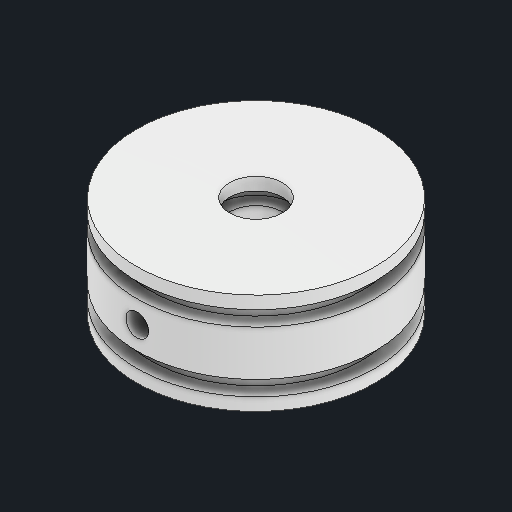
# Autodesk Inventor part: WashPiston_1
Saved by Autodesk Inventor 2024 (Build 280153000, 153)
## iProperties
Created: 2025-02-07
Part Number: WashPiston_1
Material: PVC-Piping
Document SubType Name: Modeling
Designer: Tommy Rohmann
Density: 1.4 g/cm^3
Appearance: Smooth - White
Author: Tommy Rohmann
Autodesk Inventor part; units mm, degrees
ref_plane "YZ Plane" through (0, 0, 0) normal (1, 0, 0) x (0, 1, 0)
ref_plane "XZ Plane" through (0, 0, 0) normal (0, 1, 0) x (-1, 0, 0)
ref_plane "XY Plane" through (0, 0, 0) normal (0, 0, 1) x (1, 0, 0)
sketch "WashPiston" plane through (0, 0, 0) normal (0, 0, 1) x (1, 0, 0)
  line L0 (53.5946, 10.152) -> (53.5946, 15.486)
  line L1 (53.5946, 15.486) -> (47.8796, 15.486)
  line L2 (47.8796, 15.486) -> (47.8796, 21.836)
  line L3 (47.8796, 21.836) -> (53.5946, 21.836)
  line L4 (53.5946, 21.836) -> (53.5946, 40.886)
  line L5 (53.5946, 40.886) -> (47.8796, 40.886)
  line L6 (47.8796, 40.886) -> (47.8796, 47.236)
  line L7 (47.8796, 47.236) -> (53.5946, 47.236)
  line L8 (53.5946, 47.236) -> (53.5946, 52.57)
  line L9 (54.2296, 29.069) -> (54.2296, 79.2986)
  line L10 (3.4296, 2.2226) -> (3.4296, 64.1408)
  line L11 (53.5946, 10.152) -> (3.4296, 10.152)
  line L12 (3.4296, 52.57) -> (53.5946, 52.57)
  line L13 (3.4296, 52.57) -> (3.4296, 10.152)
  line L14 (14.5421, 47.236) -> (19.8761, 47.236)
  line L15 (19.8761, 47.236) -> (19.8761, 41.902)
  line L16 (19.8761, 41.902) -> (14.5421, 41.902)
  line L17 (14.5421, 21.836) -> (3.4296, 21.836)
  line L18 (14.5421, 52.57) -> (14.5421, 47.236)
  line L19 (14.5421, 41.902) -> (14.5421, 21.836)
  point P0 (34.2963, 101.758)
  dimension "d94" = 0.635
  dimension "d95" = 6.35
  dimension "d97" = 6.35
  dimension "d98" = 19.05
  dimension "d99" = 6.35
  dimension "d100" = 5.334
  dimension "d101" = 5.334
  dimension "d103" = 5.334
  dimension "d105" = 101.6
  dimension "d108" = 22.225
  dimension "d141" = 0
  dimension "d142" = 5.334
  dimension "WashPistonHeight" = 42.418
  dimension "d431" = 30.734
  measures "d94" distance between parallel lines of L0 L9
  measures "d95" distance between parallel lines of L7 L5
  measures "d97" distance between parallel lines of L9 L6
  measures "d98" distance of L3.end L4.end
  measures "d99" distance of L1.end L2.end
  measures "d100" distance between parallel lines of L11 L1
  measures "d101" distance between parallel lines of L12 L7
  measures "d103" distance between parallel lines of L16 L14
  measures "d105" diameter of L9 L10
  measures "d108" diameter of L19 L10
  measures "d141" distance between parallel lines of L19 L18
  measures "d142" distance between parallel lines of L19 L15
  measures "WashPistonHeight" distance between parallel lines of L12 L11
  measures "d431" distance between parallel lines of L12 L17
derived "LAYOUT.ipt"
sketch "Sketch1" plane through (0, 0, 0) normal (0, 0, 1) x (1, 0, 0)
  line L0 (53.5946, 31.361) -> (3.4296, 31.361) construction
  circle A0 centre (3.4296, 31.361) radius 4.7625
  line L1 (53.5946, 10.152) -> (53.5946, 15.486)
  line L2 (53.5946, 15.486) -> (47.8796, 15.486)
  line L3 (47.8796, 15.486) -> (47.8796, 21.836)
  line L4 (47.8796, 21.836) -> (53.5946, 21.836)
  line L5 (53.5946, 21.836) -> (53.5946, 40.886)
  line L6 (53.5946, 40.886) -> (47.8796, 40.886)
  line L7 (47.8796, 40.886) -> (47.8796, 47.236)
  line L8 (47.8796, 47.236) -> (53.5946, 47.236)
  line L9 (53.5946, 47.236) -> (53.5946, 52.57)
  line L10 (54.2296, 29.069) -> (54.2296, 79.2986)
  line L11 (3.4296, 2.2226) -> (3.4296, 64.1408)
  line L12 (53.5946, 10.152) -> (3.4296, 10.152)
  line L13 (3.4296, 52.57) -> (53.5946, 52.57)
  line L14 (3.4296, 52.57) -> (3.4296, 10.152)
  line L15 (14.5421, 47.236) -> (19.8761, 47.236)
  line L16 (19.8761, 47.236) -> (19.8761, 41.902)
  line L17 (19.8761, 41.902) -> (14.5421, 41.902)
  line L18 (14.5421, 21.836) -> (3.4296, 21.836)
  line L19 (14.5421, 52.57) -> (14.5421, 47.236)
  line L20 (14.5421, 41.902) -> (14.5421, 21.836)
  point P0 (3.4296, 21.836)
  dimension "d2" = 9.525
  constraints: 2 end point, 1 centre point, 1 coincident, 2 other
  measures "d2" diameter of A0
revolve "Revolution1" add sketch "Sketch1" angle 360 about axis through (3.4296, 2.2226, 0) along (0, 1, 0) contours L18 L20 L17 L16 L15 L19 L13 L9 L8 L7 L6 L5 L4 L3 L2 L1 L12 L11
extrude "Extrusion1" cut sketch "Sketch1" along normal mid plane 161.925 contours A0 L11 | L11 A0
body "Solid1"
